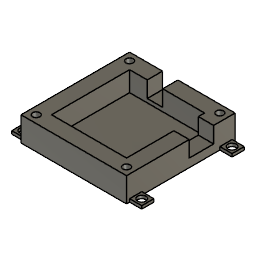
PCB_Case (Autodesk Fusion 360 archive; units mm, degrees)
design "PCB_CASE"
part number: 2026-02-23-22-04-43-512
Autodesk Fusion 360 part; units mm, degrees
sketch "Sketch1" plane through (0, 0, 0) normal (0, 0, 1) x (1, 0, 0)
  line L0 (-32.4751, 45.8669) -> (16.5249, 45.8669)
  line L1 (16.5249, 45.8669) -> (16.5249, -5.1331)
  line L2 (16.5249, -5.1331) -> (-32.4751, -5.1331)
  line L3 (-32.4751, -5.1331) -> (-32.4751, 45.8669)
  line L4 (-42.4751, 55.8669) -> (26.5249, 55.8669)
  line L5 (26.5249, 55.8669) -> (26.5249, -15.1331)
  line L6 (26.5249, -15.1331) -> (-42.4751, -15.1331)
  line L7 (-42.4751, -15.1331) -> (-42.4751, 55.8669)
  circle A0 centre (-37.4751, 50.8669) radius 2.35
  circle A1 centre (21.5249, 50.8669) radius 2.35
  circle A2 centre (-37.4751, -10.1331) radius 2.35
  circle A3 centre (21.5249, -10.1331) radius 2.35
  circle A4 centre (-37.4751, 50.8669) radius 3
  circle A5 centre (21.5249, 50.8669) radius 3
  circle A6 centre (21.5249, -10.1331) radius 3
  circle A7 centre (-37.4751, -10.1331) radius 3
  dimension "d1" = 49
  dimension "d2" = 51
  dimension "d3" = 69
  dimension "d4" = 71
  dimension "d5" = 10
  dimension "d6" = 10
  dimension "d7" = 4.7
  dimension "d8" = 4.7
  dimension "d9" = 4.7
  dimension "d10" = 4.7
  dimension "d11" = 5
  dimension "d12" = 5
  dimension "d13" = 5
  dimension "d14" = 5
  dimension "d15" = 5
  dimension "d16" = 5
  dimension "d17" = 5
  dimension "d18" = 5
  dimension "d19" = 6
  dimension "d20" = 6
  dimension "d21" = 6
  dimension "d22" = 6
  constraint horizontal L0
  constraint vertical L1
  constraint horizontal L2
  constraint vertical L3
  constraint horizontal L4
  constraint vertical L5
  constraint horizontal L6
  constraint vertical L7
  constraint concentric A0 A4
  constraint concentric A1 A5
  constraint concentric A3 A6
  constraint concentric A2 A7
  measures "d1" distance of L0.start L0.end
  measures "d2" distance of L0.start L2.end
  measures "d3" distance of L4.start L4.end
  measures "d4" distance of L4.start L6.end
  measures "d5" distance of L3 L7
  measures "d6" distance of L0 L4
  measures "d7" diameter of A0
  measures "d8" diameter of A1
  measures "d9" diameter of A2
  measures "d10" diameter of A3
  measures "d11" distance of L6 A2.centre
  measures "d12" distance of L7 A2.centre
  measures "d13" distance of L6 A3.centre
  measures "d14" distance of L5 A3.centre
  measures "d15" distance of L5 A1.centre
  measures "d16" distance of L4 A1.centre
  measures "d17" distance of L4 A0.centre
  measures "d18" distance of L7 A0.centre
  measures "d19" diameter of A4
  measures "d20" diameter of A5
  measures "d21" diameter of A6
  measures "d22" diameter of A7
extrude "Extrude1" add sketch "Sketch1" along normal blind 9.9 from surface at 3.1 contours A4 | A5 | A6 | A7 makes body 1 at (24.5211, -10.2826, 9.7) makes body 2 at (24.5211, 50.7174, 9.7) makes body 3 at (-34.4789, -10.2826, 9.7) makes body 4 at (-40.4714, 50.7174, 9.7)
extrude "Extrude2" add sketch "Sketch1" along normal blind 13 contours L4 L5 L6 L7 bodies 1 2 3 4
extrude "Extrude3" add sketch "Sketch1" along normal blind 3 contours L0 L1 L2 L3 bodies 1
sketch "Sketch2" plane through (0, 0, 13) normal (0, 0, 1) x (-1, 0, 0)
  circle A0 centre (-21.5249, 10.1331) radius 2.35
  circle A1 centre (37.4751, -50.8669) radius 2.35
  line L0 (-16.5249, 5.1331) -> (32.4751, 5.1331)
  line L1 (32.4751, 5.1331) -> (32.4751, -45.8669)
  line L2 (32.4751, -45.8669) -> (-16.5249, -45.8669)
  line L3 (-16.5249, -45.8669) -> (-16.5249, 5.1331)
  line L4 (42.4751, 15.1331) -> (-26.5249, 15.1331)
  line L5 (-26.5249, 15.1331) -> (-26.5249, -55.8669)
  line L6 (-26.5249, -55.8669) -> (42.4751, -55.8669)
  line L7 (42.4751, -55.8669) -> (42.4751, 15.1331)
  circle A2 centre (-21.5249, -50.8669) radius 2.35
  circle A3 centre (37.4751, 10.1331) radius 2.35
  line L8 (20.9211, -55.8669) -> (10.9211, -55.8669)
  line L9 (10.9211, -55.8669) -> (10.9211, -45.8669)
  line L10 (10.9211, -45.8669) -> (20.9211, -45.8669)
  line L11 (20.9211, -45.8669) -> (20.9211, -55.8669)
  line L12 (42.4751, 15.1331) -> (42.4751, -55.8669)
  line L13 (-16.5249, -41.7899) -> (-26.5249, -41.7899)
  line L14 (-26.5249, -41.7899) -> (-26.5249, -25.7899)
  line L15 (-26.5249, -25.7899) -> (-16.5249, -25.7899)
  line L16 (-16.5249, -25.7899) -> (-16.5249, -41.7899)
  line L17 (42.4751, -55.8669) -> (-26.5249, -55.8669)
  dimension "d30" = 10
  dimension "d31" = 10
  dimension "d32" = 21.554
  dimension "d33" = 10
  dimension "d34" = 16
  dimension "d35" = 14.077
  constraint horizontal L8
  constraint vertical L9
  constraint horizontal L10
  constraint vertical L11
  constraint coincident L6 L8.start
  constraint horizontal L13
  constraint vertical L14
  constraint horizontal L15
  constraint vertical L16
  constraint coincident L3 L13.start
  measures "d30" distance of L8.start L8.end
  measures "d31" distance of L8.start L10.end
  measures "d32" distance of L11 L12
  measures "d33" distance of L13.start L13.end
  measures "d34" distance of L13.start L15.end
  measures "d35" distance of L13 L17
extrude "Extrude4" cut sketch "Sketch2" against normal blind 7.5 contours L3 L5 L13 L14 L15 L16 | L2 L6 L8 L9 L10 L11 L17 bodies 1
sketch "Sketch3" plane through (0, 0, 0) normal (0, 0, 1) x (1, 0, 0)
  line L0 (-42.5221, -13.1331) -> (-50.5221, -13.1331)
  line L1 (-50.5221, -13.1331) -> (-50.5221, -5.1331)
  line L2 (-50.5221, -5.1331) -> (-42.5221, -5.1331)
  line L3 (-42.5221, -5.1331) -> (-42.5221, -13.1331)
  line L4 (26.4761, -13.1331) -> (34.4761, -13.1331)
  line L5 (34.4761, -13.1331) -> (34.4761, -5.1331)
  line L6 (34.4761, -5.1331) -> (26.4761, -5.1331)
  line L7 (26.4761, -5.1331) -> (26.4761, -13.1331)
  line L8 (26.5223, 45.8669) -> (34.5223, 45.8669)
  line L9 (34.5223, 45.8669) -> (34.5223, 53.8669)
  line L10 (34.5223, 53.8669) -> (26.5223, 53.8669)
  line L11 (26.5223, 53.8669) -> (26.5223, 45.8669)
  line L12 (-42.5, 45.8669) -> (-50.5, 45.8669)
  line L13 (-50.5, 45.8669) -> (-50.5, 53.8669)
  line L14 (-50.5, 53.8669) -> (-42.5, 53.8669)
  line L15 (-42.5, 53.8669) -> (-42.5, 45.8669)
  line L16 (26.5249, -15.1331) -> (-42.4751, -15.1331)
  line L17 (-42.4751, 55.8669) -> (26.5249, 55.8669)
  circle A0 centre (-46.5221, -9.1331) radius 2.75
  circle A1 centre (30.4761, -9.1331) radius 2.75
  circle A2 centre (30.5223, 49.8669) radius 2.75
  circle A3 centre (-46.5, 49.8669) radius 2.75
  dimension "d38" = 8
  dimension "d39" = 8
  dimension "d40" = 8
  dimension "d41" = 8
  dimension "d42" = 8
  dimension "d43" = 8
  dimension "d44" = 8
  dimension "d45" = 8
  dimension "d46" = 2
  dimension "d47" = 2
  dimension "d48" = 2
  dimension "d49" = 2
  dimension "d50" = 5.5
  dimension "d51" = 4
  dimension "d52" = 4
  dimension "d53" = 5.5
  dimension "d54" = 5.5
  dimension "d55" = 5.5
  dimension "d56" = 4
  dimension "d57" = 4
  dimension "d58" = 4
  dimension "d59" = 4
  dimension "d60" = 4
  dimension "d61" = 4
  constraint horizontal L0
  constraint vertical L1
  constraint horizontal L2
  constraint vertical L3
  constraint horizontal L4
  constraint vertical L5
  constraint horizontal L6
  constraint vertical L7
  constraint horizontal L8
  constraint vertical L9
  constraint horizontal L10
  constraint vertical L11
  constraint horizontal L12
  constraint vertical L13
  constraint horizontal L14
  constraint vertical L15
  measures "d38" distance of L0.start L0.end
  measures "d39" distance of L0.start L2.end
  measures "d40" distance of L4.start L4.end
  measures "d41" distance of L4.start L6.end
  measures "d42" distance of L8.start L8.end
  measures "d43" distance of L8.start L10.end
  measures "d44" distance of L12.start L12.end
  measures "d45" distance of L12.start L14.end
  measures "d46" distance of L0 L16
  measures "d47" distance of L4 L16
  measures "d48" distance of L10 L17
  measures "d49" distance of L14 L17
  measures "d50" diameter of A0
  measures "d51" distance of L0 A0.centre
  measures "d52" distance of L1 A0.centre
  measures "d53" diameter of A1
  measures "d54" diameter of A2
  measures "d55" diameter of A3
  measures "d56" distance of L14 A3.centre
  measures "d57" distance of L13 A3.centre
  measures "d58" distance of L10 A2.centre
  measures "d59" distance of L9 A2.centre
  measures "d60" distance of L5 A1.centre
  measures "d61" distance of L4 A1.centre
extrude "Extrude5" add sketch "Sketch3" along normal blind 2 bodies 1 makes body 5 at (-46.5685, 53.4477, 0) makes body 6 at (-46.4536, -12.7138, 0)
extrude "Extrude6" add 2 faces at (19.8582, 15.4823, 13) (-1.7725, 49.2003, 13) along direction (0, 0, 1) blind 2 on bodies 1 bodies 1
extrude "Extrude7" add 2 faces at (19.8582, 15.4823, 15) (-1.7725, 49.2003, 15) along direction (0, 0, 1) blind 1 on bodies 1 bodies 1

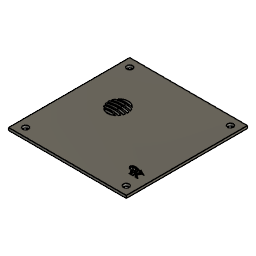
design "PCB_TOP"
part number: 2026-02-23-22-28-18-651
Autodesk Fusion 360 part; units mm, degrees
sketch "Sketch1" plane through (0, 0, 0) normal (0, 0, 1) x (1, 0, 0)
  line L0 (-55.9108, 58.924) -> (13.0892, 58.924)
  line L1 (13.0892, 58.924) -> (13.0892, -12.076)
  line L2 (13.0892, -12.076) -> (-55.9108, -12.076)
  line L3 (-55.9108, -12.076) -> (-55.9108, 58.924)
  circle A0 centre (-50.9108, 53.924) radius 1.7
  circle A1 centre (8.0892, 53.924) radius 1.7
  circle A2 centre (-50.9108, -7.076) radius 1.7
  circle A3 centre (8.0892, -7.076) radius 1.7
  dimension "d1" = 69
  dimension "d2" = 71
  dimension "d3" = 3.4
  dimension "d4" = 3.4
  dimension "d5" = 3.4
  dimension "d6" = 3.4
  dimension "d7" = 5
  dimension "d8" = 5
  dimension "d9" = 5
  dimension "d10" = 5
  dimension "d11" = 5
  dimension "d12" = 5
  dimension "d13" = 5
  dimension "d14" = 5
  constraint horizontal L0
  constraint vertical L1
  constraint horizontal L2
  constraint vertical L3
  measures "d1" distance of L0.start L0.end
  measures "d2" distance of L0.start L2.end
  measures "d3" diameter of A0
  measures "d4" diameter of A1
  measures "d5" diameter of A2
  measures "d6" diameter of A3
  measures "d7" distance of L0 A0.centre
  measures "d8" distance of L3 A0.centre
  measures "d9" distance of L0 A1.centre
  measures "d10" distance of L1 A1.centre
  measures "d11" distance of L2 A2.centre
  measures "d12" distance of L3 A2.centre
  measures "d13" distance of L1 A3.centre
  measures "d14" distance of L2 A3.centre
extrude "Extrude1" add sketch "Sketch1" along normal blind 1.5
sketch "Sketch2" plane through (0, 0, 0) normal (0, 0, -1) x (1, 0, 0)
  circle A0 centre (-50.9108, -53.924) radius 1.7
  circle A1 centre (-50.9108, 7.076) radius 1.7
  circle A2 centre (8.0892, 7.076) radius 1.7
  circle A3 centre (8.0892, -53.924) radius 1.7
  line L0 (13.0892, 12.076) -> (-55.9108, 12.076)
  line L1 (-55.9108, 12.076) -> (-55.9108, -58.924)
  line L2 (-55.9108, -58.924) -> (13.0892, -58.924)
  line L3 (13.0892, -58.924) -> (13.0892, 12.076)
sketch "Sketch3" plane through (0, 0, 0) normal (0, 0, -1) x (1, 0, 0)
sketch "Sketch4" plane through (0, 0, 0) normal (0, 0, 1) x (1, 0, 0)
  spline S0 degree 3 poles (5.6281, 1.7474) (5.8196, 2.0554) (6.0075, 2.3594) (6.1973, 2.6623) (6.3487, 2.9041) (6.502, 3.1447) (6.656, 3.3849) knots 0 0 0 0 1 1 1 2 2 2 2
  spline S1 degree 3 poles (6.656, 3.3849) (6.6671, 3.4022) (6.692, 3.4235) (6.7087, 3.422) knots 2 2 2 2 3 3 3 3
  spline S2 degree 3 poles (6.7087, 3.422) (6.7689, 3.4166) (6.8284, 3.4023) (6.9022, 3.3887) knots 3 3 3 3 4 4 4 4
  line L0 (6.9022, 3.3887) -> (5.6608, 1.7184)
  line L1 (5.6608, 1.7184) -> (5.6281, 1.7474)
  line L2 (4.5804, 1.7909) -> (4.5624, 1.7702)
  line L3 (4.5624, 1.7702) -> (5.8909, 0.5262)
  line L4 (5.8909, 0.5262) -> (5.8872, 0.5223)
  line L5 (5.8872, 0.5223) -> (4.6487, 1.4888)
  spline S3 degree 3 poles (4.6487, 1.4888) (4.6512, 1.4764) (4.6534, 1.4612) (4.6573, 1.4465) (4.7531, 1.0839) (4.8509, 0.7218) (4.9442, 0.3586) (4.9738, 0.2436) (5.0121, 0.1286) (5, 0) knots 4 4 4 4 5 5 5 6 6 6 7 7 7 7
  spline S4 degree 3 poles (5, 0) (4.9265, 0.0282) (4.8723, 0.0673) (4.8514, 0.146) (4.7035, 0.7025) (4.5538, 1.2585) (4.4057, 1.815) (4.2636, 2.3493) (4.1247, 2.8845) (3.9798, 3.4181) (3.9538, 3.5138) (3.9711, 3.5848) (4.0485, 3.6489) knots 7 7 7 7 8 8 8 9 9 9 10 10 10 11 11 11 11
  spline S5 degree 3 poles (4.0485, 3.6489) (4.057, 3.6244) (4.0653, 3.6032) (4.0716, 3.5815) (4.1522, 3.306) (4.2349, 3.0312) (4.3114, 2.7546) (4.3374, 2.6606) (4.3738, 2.584) (4.4575, 2.5237) (4.5786, 2.4365) (4.6889, 2.3342) (4.8053, 2.2373) knots 11 11 11 11 12 12 12 13 13 13 14 14 14 15 15 15 15
  line L6 (4.8053, 2.2373) -> (5.6163, 3.6354)
  line L7 (5.6163, 3.6354) -> (6.5426, 3.4546)
  line L8 (6.5426, 3.4546) -> (5.4688, 1.7209)
  spline S6 degree 3 poles (5.4688, 1.7209) (5.4886, 1.7024) (5.5045, 1.6858) (5.522, 1.6712) (5.9169, 1.3412) (6.3108, 1.0098) (6.7075, 0.682) (7.0163, 0.4267) (7.3347, 0.1848) (7.7042, 0.0204) knots 18 18 18 18 19 19 19 20 20 20 21 21 21 21
  spline S7 degree 3 poles (7.7042, 0.0204) (7.7072, 0.0191) (7.7082, 0.0133) (7.7106, 0.0087) knots 21 21 21 21 22 22 22 22
  line L9 (7.7106, 0.0087) -> (6.141, 0.0087)
  spline S8 degree 3 poles (6.141, 0.0087) (6.2596, 0.0588) (6.3866, 0.066) (6.4574, 0.1898) knots 23 23 23 23 24 24 24 24
  line L10 (6.4574, 0.1898) -> (4.5804, 1.7909)
  line L11 (3.5521, 4.7959) -> (3.5501, 4.7818)
  spline S9 degree 3 poles (3.5501, 4.7818) (3.5432, 4.7818) (3.5362, 4.7808) (3.5295, 4.782) (3.3494, 4.8151) (3.1703, 4.8556) (2.9891, 4.8801) (2.703, 4.9188) (2.4161, 4.9559) (2.1284, 4.9765) (1.9076, 4.9923) (1.6849, 4.9868) (1.4633, 4.9816) (1.1041, 4.9731) (0.7512, 4.9194) (0.4077, 4.8114) (0.1446, 4.7288) (-0.1029, 4.6155) (-0.3041, 4.4211) (-0.4819, 4.2492) (-0.586, 4.0442) (-0.565, 3.7891) (-0.5636, 3.7712) (-0.5588, 3.7537) (-0.5556, 3.736) knots 1 1 1 1 2 2 2 3 3 3 4 4 4 5 5 5 6 6 6 7 7 7 8 8 8 9 9 9 9
  spline S10 degree 3 poles (-0.5556, 3.736) (-0.5472, 3.9502) (-0.4576, 4.1249) (-0.3145, 4.276) (-0.121, 4.4805) (0.1241, 4.5996) (0.3866, 4.6832) (0.8641, 4.8353) (1.3569, 4.8719) (1.8545, 4.8528) (2.3079, 4.8355) (2.7558, 4.7693) (3.2, 4.6793) (3.7596, 4.5658) (4.3094, 4.414) (4.8543, 4.244) (4.9709, 4.2076) (5.0879, 4.1724) (5.2047, 4.1367) knots 9 9 9 9 10 10 10 11 11 11 12 12 12 13 13 13 14 14 14 15 15 15 15
  line L12 (5.2047, 4.1367) -> (5.2091, 4.1476)
  line L13 (5.2091, 4.1476) -> (3.9846, 4.702)
  spline S11 degree 3 poles (3.9846, 4.702) (4.577, 4.5581) (5.1429, 4.3403) (5.7082, 4.0808) knots 17 17 17 17 18 18 18 18
  spline S12 degree 3 poles (5.7082, 4.0808) (5.4595, 4.2577) (5.2178, 4.4195) (4.9875, 4.5961) (4.7566, 4.7731) (4.537, 4.965) (4.3124, 5.1503) knots 18 18 18 18 19 19 19 20 20 20 20
  line L14 (4.3124, 5.1503) -> (4.3217, 5.1631)
  spline S13 degree 3 poles (4.3217, 5.1631) (5.5089, 4.473) (6.7466, 3.8854) (8.0084, 3.3461) knots 21 21 21 21 22 22 22 22
  spline S14 degree 3 poles (8.0084, 3.3461) (7.662, 3.4033) (7.3162, 3.4598) (6.9722, 3.5253) (6.261, 3.6607) (5.5513, 3.8039) (4.8399, 3.9379) (4.3277, 4.0343) (3.8146, 4.1272) (3.3001, 4.2106) (2.7534, 4.2992) (2.2027, 4.345) (1.6475, 4.3283) (1.3737, 4.3201) (1.1022, 4.2966) (0.8346, 4.2389) (0.5729, 4.1826) (0.3217, 4.0989) (0.104, 3.9348) (-0.1303, 3.7584) (-0.2087, 3.495) (-0.1029, 3.2211) (-0.0226, 3.0131) (0.1228, 2.8533) (0.2889, 2.7107) (0.3566, 2.6525) (0.428, 2.5988) (0.4978, 2.5431) knots 22 22 22 22 23 23 23 24 24 24 25 25 25 26 26 26 27 27 27 28 28 28 29 29 29 30 30 30 31 31 31 31
  spline S15 degree 3 poles (0.4978, 2.5431) (0.2478, 2.6652) (0.0143, 2.8111) (-0.1869, 3.0047) (-0.3924, 3.2026) (-0.5444, 3.435) (-0.6323, 3.7066) (-0.7351, 4.0241) (-0.6754, 4.3114) (-0.4598, 4.566) (-0.3004, 4.7543) (-0.0926, 4.8718) (0.1325, 4.9605) (0.6054, 5.1469) (1.0996, 5.1935) (1.6022, 5.1694) (2.0538, 5.1477) (2.4991, 5.0781) (2.9369, 4.9649) (3.1428, 4.9117) (3.3471, 4.8524) (3.5521, 4.7959) knots 31 31 31 31 32 32 32 33 33 33 34 34 34 35 35 35 36 36 36 37 37 37 38 38 38 38
  spline S16 degree 3 poles (3.0792, 2.6831) (3.0761, 2.705) (3.0755, 2.7171) (3.0725, 2.7285) (2.998, 3.0093) (2.9217, 3.2897) (2.8492, 3.571) (2.8121, 3.7152) (2.7298, 3.8241) (2.6093, 3.9072) (2.5961, 3.9164) (2.5839, 3.9269) (2.5627, 3.9435) knots 0 0 0 0 1 1 1 2 2 2 3 3 3 4 4 4 4
  spline S17 degree 3 poles (2.5627, 3.9435) (2.5819, 3.9435) (2.5886, 3.9436) (2.5952, 3.9435) (2.8859, 3.9363) (3.1765, 3.931) (3.4671, 3.9211) (3.5886, 3.9169) (3.7097, 3.9033) (3.8222, 3.8498) (3.8726, 3.8257) (3.9161, 3.7951) (3.9397, 3.7398) knots 4 4 4 4 5 5 5 6 6 6 7 7 7 8 8 8 8
  spline S18 degree 3 poles (3.9397, 3.7398) (3.8168, 3.6538) (3.7944, 3.5454) (3.8344, 3.4021) (3.9736, 2.9036) (4.1027, 2.4022) (4.2364, 1.9021) (4.4001, 1.2897) (4.5646, 0.6775) (4.7287, 0.0652) (4.7334, 0.0475) (4.7365, 0.0294) (4.7407, 0.01) knots 8 8 8 8 9 9 9 10 10 10 11 11 11 12 12 12 12
  line L15 (4.7407, 0.01) -> (2.6293, 0.01)
  spline S19 degree 3 poles (2.6293, 0.01) (2.7311, 0.0489) (2.8207, 0.0792) (2.9069, 0.1171) (2.9939, 0.1554) (3.0751, 0.2044) (3.1385, 0.2849) knots 13 13 13 13 14 14 14 15 15 15 15
  spline S20 degree 3 poles (3.1385, 0.2849) (2.6116, 0.9618) (2.0699, 1.623) (1.5036, 2.2696) knots 15 15 15 15 16 16 16 16
  spline S21 degree 3 poles (1.5036, 2.2696) (1.5146, 2.2711) (1.5184, 2.2727) (1.5212, 2.2717) knots 16 16 16 16 17 17 17 17
  spline S22 degree 3 poles (1.5212, 2.2717) (1.8422, 2.158) (2.1718, 2.0759) (2.5055, 2.0097) (2.5464, 2.0016) (2.5744, 1.984) (2.5995, 1.9511) (2.9298, 1.5179) (3.2612, 1.0856) (3.5924, 0.6531) (3.6084, 0.6323) (3.6246, 0.6118) (3.6481, 0.5815) knots 17 17 17 17 18 18 18 19 19 19 20 20 20 21 21 21 21
  spline S23 degree 3 poles (3.6481, 0.5815) (3.6467, 0.601) (3.6472, 0.6063) (3.6459, 0.6112) (3.5264, 1.044) (3.4064, 1.4768) (3.2873, 1.9097) (3.2555, 2.025) (3.2565, 2.0238) (3.135, 2.0402) (2.6367, 2.1074) (2.1447, 2.2049) (1.6647, 2.3568) (1.3092, 2.4693) (0.9646, 2.6068) (0.6529, 2.816) (0.5076, 2.9135) (0.3678, 3.0185) (0.2641, 3.1624) (0.139, 3.3361) (0.0847, 3.5235) (0.1843, 3.7274) (0.3644, 4.0959) (0.9086, 4.1348) (1.1664, 3.7998) (1.3084, 3.6154) (1.4505, 3.4311) (1.5914, 3.246) (1.6369, 3.1862) (1.6863, 3.1346) (1.7602, 3.1086) (2.054, 3.0053) (2.3457, 2.8958) (2.641, 2.7969) (2.7817, 2.7498) (2.9286, 2.7215) (3.0792, 2.6831) knots 21 21 21 21 22 22 22 23 23 23 24 24 24 25 25 25 26 26 26 27 27 27 28 28 28 29 29 29 30 30 30 31 31 31 32 32 32 33 33 33 33
  line L16 (3.7963, 2.3959) -> (3.7953, 2.3879)
  spline S24 degree 3 poles (3.7953, 2.3879) (3.7747, 2.3879) (3.754, 2.3863) (3.7335, 2.3882) (3.5881, 2.4016) (3.4419, 2.4105) (3.2974, 2.4308) (2.7728, 2.5044) (2.2593, 2.6253) (1.7634, 2.8135) (1.4001, 2.9513) (1.0496, 3.1153) (0.7397, 3.3549) (0.6837, 3.3982) (0.6294, 3.4437) (0.5744, 3.4881) knots 1 1 1 1 2 2 2 3 3 3 4 4 4 5 5 5 6 6 6 6
  spline S25 degree 3 poles (0.5744, 3.4881) (0.5844, 3.4935) (0.5891, 3.4922) (0.593, 3.4895) knots 6 6 6 6 7 7 7 7
  spline S26 degree 3 poles (0.593, 3.4895) (0.8417, 3.32) (1.1118, 3.1913) (1.3895, 3.0786) (2.0638, 2.8049) (2.7634, 2.6158) (3.4734, 2.4622) (3.5808, 2.439) (3.6886, 2.4179) (3.7963, 2.3959) knots 7 7 7 7 8 8 8 9 9 9 10 10 10 10
  spline S27 degree 3 poles (3.0792, 2.6831) (2.9286, 2.7215) (2.7817, 2.7498) (2.641, 2.7969) (2.3457, 2.8958) (2.054, 3.0053) (1.7602, 3.1086) (1.6863, 3.1346) (1.6369, 3.1862) (1.5914, 3.246) (1.4505, 3.4311) (1.3084, 3.6154) (1.1664, 3.7998) (0.9086, 4.1348) (0.3644, 4.0959) (0.1843, 3.7274) (0.0847, 3.5235) (0.139, 3.3361) (0.2641, 3.1624) (0.3678, 3.0185) (0.5076, 2.9135) (0.6529, 2.816) (0.9646, 2.6068) (1.3092, 2.4693) (1.6647, 2.3568) (2.1447, 2.2049) (2.6367, 2.1074) (3.135, 2.0402) (3.2565, 2.0238) (3.2555, 2.025) (3.2873, 1.9097) (3.4064, 1.4768) (3.5264, 1.044) (3.6459, 0.6112) (3.6472, 0.6063) (3.6467, 0.601) (3.6481, 0.5815) knots 0 0 0 0 1 1 1 2 2 2 3 3 3 4 4 4 5 5 5 6 6 6 7 7 7 8 8 8 9 9 9 10 10 10 11 11 11 12 12 12 12
  spline S28 degree 3 poles (3.6481, 0.5815) (3.6246, 0.6118) (3.6084, 0.6323) (3.5924, 0.6531) (3.2612, 1.0856) (2.9298, 1.5179) (2.5995, 1.9511) (2.5744, 1.984) (2.5464, 2.0016) (2.5055, 2.0097) (2.1718, 2.0759) (1.8422, 2.158) (1.5212, 2.2717) knots 12 12 12 12 13 13 13 14 14 14 15 15 15 16 16 16 16
  spline S29 degree 3 poles (1.5212, 2.2717) (1.5184, 2.2727) (1.5146, 2.2711) (1.5036, 2.2696) knots 16 16 16 16 17 17 17 17
  spline S30 degree 3 poles (1.5036, 2.2696) (2.0699, 1.623) (2.6116, 0.9618) (3.1385, 0.2849) knots 17 17 17 17 18 18 18 18
  spline S31 degree 3 poles (3.1385, 0.2849) (3.0751, 0.2044) (2.9939, 0.1554) (2.9069, 0.1171) (2.8207, 0.0792) (2.7311, 0.0489) (2.6293, 0.01) knots 18 18 18 18 19 19 19 20 20 20 20
  line L17 (2.6293, 0.01) -> (4.7407, 0.01)
  spline S32 degree 3 poles (4.7407, 0.01) (4.7365, 0.0294) (4.7334, 0.0475) (4.7287, 0.0652) (4.5646, 0.6775) (4.4001, 1.2897) (4.2364, 1.9021) (4.1027, 2.4022) (3.9736, 2.9036) (3.8344, 3.4021) (3.7944, 3.5454) (3.8168, 3.6538) (3.9397, 3.7398) knots 21 21 21 21 22 22 22 23 23 23 24 24 24 25 25 25 25
  spline S33 degree 3 poles (3.9397, 3.7398) (3.9161, 3.7951) (3.8726, 3.8257) (3.8222, 3.8498) (3.7097, 3.9033) (3.5886, 3.9169) (3.4671, 3.9211) (3.1765, 3.931) (2.8859, 3.9363) (2.5952, 3.9435) (2.5886, 3.9436) (2.5819, 3.9435) (2.5627, 3.9435) knots 25 25 25 25 26 26 26 27 27 27 28 28 28 29 29 29 29
  spline S34 degree 3 poles (2.5627, 3.9435) (2.5839, 3.9269) (2.5961, 3.9164) (2.6093, 3.9072) (2.7298, 3.8241) (2.8121, 3.7152) (2.8492, 3.571) (2.9217, 3.2897) (2.998, 3.0093) (3.0725, 2.7285) (3.0755, 2.7171) (3.0761, 2.705) (3.0792, 2.6831) knots 29 29 29 29 30 30 30 31 31 31 32 32 32 33 33 33 33
  spline S35 degree 3 poles (3.5521, 4.7959) (3.3471, 4.8524) (3.1428, 4.9117) (2.9369, 4.9649) (2.4991, 5.0781) (2.0538, 5.1477) (1.6022, 5.1694) (1.0996, 5.1935) (0.6054, 5.1469) (0.1325, 4.9605) (-0.0926, 4.8718) (-0.3004, 4.7543) (-0.4598, 4.566) (-0.6754, 4.3114) (-0.7351, 4.0241) (-0.6323, 3.7066) (-0.5444, 3.435) (-0.3924, 3.2026) (-0.1869, 3.0047) (0.0143, 2.8111) (0.2478, 2.6652) (0.4978, 2.5431) knots 0 0 0 0 1 1 1 2 2 2 3 3 3 4 4 4 5 5 5 6 6 6 7 7 7 7
  spline S36 degree 3 poles (0.4978, 2.5431) (0.428, 2.5988) (0.3566, 2.6525) (0.2889, 2.7107) (0.1228, 2.8533) (-0.0226, 3.0131) (-0.1029, 3.2211) (-0.2087, 3.495) (-0.1303, 3.7584) (0.104, 3.9348) (0.3217, 4.0989) (0.5729, 4.1826) (0.8346, 4.2389) (1.1022, 4.2966) (1.3737, 4.3201) (1.6475, 4.3283) (2.2027, 4.345) (2.7534, 4.2992) (3.3001, 4.2106) (3.8146, 4.1272) (4.3277, 4.0343) (4.8399, 3.9379) (5.5513, 3.8039) (6.261, 3.6607) (6.9722, 3.5253) (7.3162, 3.4598) (7.662, 3.4033) (8.0084, 3.3461) knots 7 7 7 7 8 8 8 9 9 9 10 10 10 11 11 11 12 12 12 13 13 13 14 14 14 15 15 15 16 16 16 16
  spline S37 degree 3 poles (8.0084, 3.3461) (6.7466, 3.8854) (5.5089, 4.473) (4.3217, 5.1631) knots 16 16 16 16 17 17 17 17
  line L18 (4.3217, 5.1631) -> (4.3124, 5.1503)
  spline S38 degree 3 poles (4.3124, 5.1503) (4.537, 4.965) (4.7566, 4.7731) (4.9875, 4.5961) (5.2178, 4.4195) (5.4595, 4.2577) (5.7082, 4.0808) knots 18 18 18 18 19 19 19 20 20 20 20
  spline S39 degree 3 poles (5.7082, 4.0808) (5.1429, 4.3403) (4.577, 4.5581) (3.9846, 4.702) knots 20 20 20 20 21 21 21 21
  line L19 (3.9846, 4.702) -> (5.2091, 4.1476)
  line L20 (5.2091, 4.1476) -> (5.2047, 4.1367)
  spline S40 degree 3 poles (5.2047, 4.1367) (5.0879, 4.1724) (4.9709, 4.2076) (4.8543, 4.244) (4.3094, 4.414) (3.7596, 4.5658) (3.2, 4.6793) (2.7558, 4.7693) (2.3079, 4.8355) (1.8545, 4.8528) (1.3569, 4.8719) (0.8641, 4.8353) (0.3866, 4.6832) (0.1241, 4.5996) (-0.121, 4.4805) (-0.3145, 4.276) (-0.4576, 4.1249) (-0.5472, 3.9502) (-0.5556, 3.736) knots 23 23 23 23 24 24 24 25 25 25 26 26 26 27 27 27 28 28 28 29 29 29 29
  spline S41 degree 3 poles (-0.5556, 3.736) (-0.5588, 3.7537) (-0.5636, 3.7712) (-0.565, 3.7891) (-0.586, 4.0442) (-0.4819, 4.2492) (-0.3041, 4.4211) (-0.1029, 4.6155) (0.1446, 4.7288) (0.4077, 4.8114) (0.7512, 4.9194) (1.1041, 4.9731) (1.4633, 4.9816) (1.6849, 4.9868) (1.9076, 4.9923) (2.1284, 4.9765) (2.4161, 4.9559) (2.703, 4.9188) (2.9891, 4.8801) (3.1703, 4.8556) (3.3494, 4.8151) (3.5295, 4.782) (3.5362, 4.7808) (3.5432, 4.7818) (3.5501, 4.7818) knots 29 29 29 29 30 30 30 31 31 31 32 32 32 33 33 33 34 34 34 35 35 35 36 36 36 37 37 37 37
  line L21 (3.5501, 4.7818) -> (3.5521, 4.7959)
  line L22 (4.5804, 1.7909) -> (6.4574, 0.1898)
  spline S42 degree 3 poles (6.4574, 0.1898) (6.3866, 0.066) (6.2596, 0.0588) (6.141, 0.0087) knots 1 1 1 1 2 2 2 2
  line L23 (6.141, 0.0087) -> (7.7106, 0.0087)
  spline S43 degree 3 poles (7.7106, 0.0087) (7.7082, 0.0133) (7.7072, 0.0191) (7.7042, 0.0204) knots 3 3 3 3 4 4 4 4
  spline S44 degree 3 poles (7.7042, 0.0204) (7.3347, 0.1848) (7.0163, 0.4267) (6.7075, 0.682) (6.3108, 1.0098) (5.9169, 1.3412) (5.522, 1.6712) (5.5045, 1.6858) (5.4886, 1.7024) (5.4688, 1.7209) knots 4 4 4 4 5 5 5 6 6 6 7 7 7 7
  line L24 (5.4688, 1.7209) -> (6.5426, 3.4546)
  line L25 (6.5426, 3.4546) -> (5.6163, 3.6354)
  line L26 (5.6163, 3.6354) -> (4.8053, 2.2373)
  spline S45 degree 3 poles (4.8053, 2.2373) (4.6889, 2.3342) (4.5786, 2.4365) (4.4575, 2.5237) (4.3738, 2.584) (4.3374, 2.6606) (4.3114, 2.7546) (4.2349, 3.0312) (4.1522, 3.306) (4.0716, 3.5815) (4.0653, 3.6032) (4.057, 3.6244) (4.0485, 3.6489) knots 10 10 10 10 11 11 11 12 12 12 13 13 13 14 14 14 14
  spline S46 degree 3 poles (4.0485, 3.6489) (3.9711, 3.5848) (3.9538, 3.5138) (3.9798, 3.4181) (4.1247, 2.8845) (4.2636, 2.3493) (4.4057, 1.815) (4.5538, 1.2585) (4.7035, 0.7025) (4.8514, 0.146) (4.8723, 0.0673) (4.9265, 0.0282) (5, 0) knots 14 14 14 14 15 15 15 16 16 16 17 17 17 18 18 18 18
  spline S47 degree 3 poles (5, 0) (5.0121, 0.1286) (4.9738, 0.2436) (4.9442, 0.3586) (4.8509, 0.7218) (4.7531, 1.0839) (4.6573, 1.4465) (4.6534, 1.4612) (4.6512, 1.4764) (4.6487, 1.4888) knots 18 18 18 18 19 19 19 20 20 20 21 21 21 21
  line L27 (4.6487, 1.4888) -> (5.8872, 0.5223)
  line L28 (5.8872, 0.5223) -> (5.8909, 0.5262)
  line L29 (5.8909, 0.5262) -> (4.5624, 1.7702)
  line L30 (4.5624, 1.7702) -> (4.5804, 1.7909)
  line L31 (5.6281, 1.7474) -> (5.6608, 1.7184)
  line L32 (5.6608, 1.7184) -> (6.9022, 3.3887)
  spline S48 degree 3 poles (6.9022, 3.3887) (6.8284, 3.4023) (6.7689, 3.4166) (6.7087, 3.422) knots 2 2 2 2 3 3 3 3
  spline S49 degree 3 poles (6.7087, 3.422) (6.692, 3.4235) (6.6671, 3.4022) (6.656, 3.3849) knots 3 3 3 3 4 4 4 4
  spline S50 degree 3 poles (6.656, 3.3849) (6.502, 3.1447) (6.3487, 2.9041) (6.1973, 2.6623) (6.0075, 2.3594) (5.8196, 2.0554) (5.6281, 1.7474) knots 4 4 4 4 5 5 5 6 6 6 6
  spline S51 degree 3 poles (3.7963, 2.3959) (3.6886, 2.4179) (3.5808, 2.439) (3.4734, 2.4622) (2.7634, 2.6158) (2.0638, 2.8049) (1.3895, 3.0786) (1.1118, 3.1913) (0.8417, 3.32) (0.593, 3.4895) knots 0 0 0 0 1 1 1 2 2 2 3 3 3 3
  spline S52 degree 3 poles (0.593, 3.4895) (0.5891, 3.4922) (0.5844, 3.4935) (0.5744, 3.4881) knots 3 3 3 3 4 4 4 4
  spline S53 degree 3 poles (0.5744, 3.4881) (0.6294, 3.4437) (0.6837, 3.3982) (0.7397, 3.3549) (1.0496, 3.1153) (1.4001, 2.9513) (1.7634, 2.8135) (2.2593, 2.6253) (2.7728, 2.5044) (3.2974, 2.4308) (3.4419, 2.4105) (3.5881, 2.4016) (3.7335, 2.3882) (3.754, 2.3863) (3.7747, 2.3879) (3.7953, 2.3879) knots 4 4 4 4 5 5 5 6 6 6 7 7 7 8 8 8 9 9 9 9
  line L33 (3.7953, 2.3879) -> (3.7963, 2.3959)
extrude "Extrude2" cut sketch "Sketch4" along normal blind 1.5 contours S0 S1 S2 L0 L1 L31 L32 S48 S49 S50 | L2 L3 L4 L5 S3 S4 S5 L6 L7 L8 S6 S7 L9 S8 L10 L22 S42 L23 S43 S44 L24 L25 L26 S45 S46 S47 L27 L28 L29 L30 | L11 S9 S10 L12 L13 S11 S12 L14 S13 S14 S15 S35 S36 S37 L18 S38 S39 L19 L20 S40 S41 L21 | S16 S17 S18 L15 S19 S20 S21 S22 S23 S27 S28 S29 S30 S31 L17 S32 S33 S34 | L16 S24 S25 S26 S51 S52 S53 L33
sketch "Sketch6" plane through (0, 0, 0) normal (0, 0, -1) x (1, 0, 0)
  line L0 (5.8909, -0.5262) -> (4.5624, -1.7702)
  line L1 (4.5624, -1.7702) -> (4.5804, -1.7909)
  line L2 (4.5804, -1.7909) -> (6.4574, -0.1898)
  spline S0 degree 3 poles (6.4574, -0.1898) (6.3866, -0.066) (6.2596, -0.0588) (6.141, -0.0087) knots 1 1 1 1 2 2 2 2
  line L3 (6.141, -0.0087) -> (7.7106, -0.0087)
  spline S1 degree 3 poles (7.7106, -0.0087) (7.7082, -0.0133) (7.7072, -0.0191) (7.7042, -0.0204) knots 3 3 3 3 4 4 4 4
  spline S2 degree 3 poles (7.7042, -0.0204) (7.3347, -0.1848) (7.0163, -0.4267) (6.7075, -0.682) (6.3108, -1.0098) (5.9169, -1.3412) (5.522, -1.6712) (5.5045, -1.6858) (5.4886, -1.7024) (5.4688, -1.7209) knots 4 4 4 4 5 5 5 6 6 6 7 7 7 7
  line L4 (5.4688, -1.7209) -> (6.5426, -3.4546)
  line L5 (6.5426, -3.4546) -> (5.6163, -3.6354)
  line L6 (5.6163, -3.6354) -> (4.8053, -2.2373)
  spline S3 degree 3 poles (4.8053, -2.2373) (4.6889, -2.3342) (4.5786, -2.4365) (4.4575, -2.5237) (4.3738, -2.584) (4.3374, -2.6606) (4.3114, -2.7546) (4.2349, -3.0312) (4.1522, -3.306) (4.0716, -3.5815) (4.0653, -3.6032) (4.057, -3.6244) (4.0485, -3.6489) knots 10 10 10 10 11 11 11 12 12 12 13 13 13 14 14 14 14
  spline S4 degree 3 poles (4.0485, -3.6489) (3.9711, -3.5848) (3.9538, -3.5138) (3.9798, -3.4181) (4.1247, -2.8845) (4.2636, -2.3493) (4.4057, -1.815) (4.5538, -1.2585) (4.7035, -0.7025) (4.8514, -0.146) (4.8723, -0.0673) (4.9265, -0.0282) (5, 0) knots 14 14 14 14 15 15 15 16 16 16 17 17 17 18 18 18 18
  spline S5 degree 3 poles (5, 0) (5.0121, -0.1286) (4.9738, -0.2436) (4.9442, -0.3586) (4.8509, -0.7218) (4.7531, -1.0839) (4.6573, -1.4465) (4.6534, -1.4612) (4.6512, -1.4764) (4.6487, -1.4888) knots 18 18 18 18 19 19 19 20 20 20 21 21 21 21
  line L7 (4.6487, -1.4888) -> (5.8872, -0.5223)
  line L8 (5.8872, -0.5223) -> (5.8909, -0.5262)
  spline S6 degree 3 poles (-0.5556, -3.736) (-0.5588, -3.7537) (-0.5636, -3.7712) (-0.565, -3.7891) (-0.586, -4.0442) (-0.4819, -4.2492) (-0.3041, -4.4211) (-0.1029, -4.6155) (0.1446, -4.7288) (0.4077, -4.8114) (0.7512, -4.9194) (1.1041, -4.9731) (1.4633, -4.9816) (1.6849, -4.9868) (1.9076, -4.9923) (2.1284, -4.9765) (2.4161, -4.9559) (2.703, -4.9188) (2.9891, -4.8801) (3.1703, -4.8556) (3.3494, -4.8151) (3.5295, -4.782) (3.5362, -4.7808) (3.5432, -4.7818) (3.5501, -4.7818) knots 29 29 29 29 30 30 30 31 31 31 32 32 32 33 33 33 34 34 34 35 35 35 36 36 36 37 37 37 37
  line L9 (3.5501, -4.7818) -> (3.5521, -4.7959)
  spline S7 degree 3 poles (3.5521, -4.7959) (3.3471, -4.8524) (3.1428, -4.9117) (2.9369, -4.9649) (2.4991, -5.0781) (2.0538, -5.1477) (1.6022, -5.1694) (1.0996, -5.1935) (0.6054, -5.1469) (0.1325, -4.9605) (-0.0926, -4.8718) (-0.3004, -4.7543) (-0.4598, -4.566) (-0.6754, -4.3114) (-0.7351, -4.0241) (-0.6323, -3.7066) (-0.5444, -3.435) (-0.3924, -3.2026) (-0.1869, -3.0047) (0.0143, -2.8111) (0.2478, -2.6652) (0.4978, -2.5431) knots 0 0 0 0 1 1 1 2 2 2 3 3 3 4 4 4 5 5 5 6 6 6 7 7 7 7
  spline S8 degree 3 poles (0.4978, -2.5431) (0.428, -2.5988) (0.3566, -2.6525) (0.2889, -2.7107) (0.1228, -2.8533) (-0.0226, -3.0131) (-0.1029, -3.2211) (-0.2087, -3.495) (-0.1303, -3.7584) (0.104, -3.9348) (0.3217, -4.0989) (0.5729, -4.1826) (0.8346, -4.2389) (1.1022, -4.2966) (1.3737, -4.3201) (1.6475, -4.3283) (2.2027, -4.345) (2.7534, -4.2992) (3.3001, -4.2106) (3.8146, -4.1272) (4.3277, -4.0343) (4.8399, -3.9379) (5.5513, -3.8039) (6.261, -3.6607) (6.9722, -3.5253) (7.3162, -3.4598) (7.662, -3.4033) (8.0084, -3.3461) knots 7 7 7 7 8 8 8 9 9 9 10 10 10 11 11 11 12 12 12 13 13 13 14 14 14 15 15 15 16 16 16 16
  spline S9 degree 3 poles (8.0084, -3.3461) (6.7466, -3.8854) (5.5089, -4.473) (4.3217, -5.1631) knots 16 16 16 16 17 17 17 17
  line L10 (4.3217, -5.1631) -> (4.3124, -5.1503)
  spline S10 degree 3 poles (4.3124, -5.1503) (4.537, -4.965) (4.7566, -4.7731) (4.9875, -4.5961) (5.2178, -4.4195) (5.4595, -4.2577) (5.7082, -4.0808) knots 18 18 18 18 19 19 19 20 20 20 20
  spline S11 degree 3 poles (5.7082, -4.0808) (5.1429, -4.3403) (4.577, -4.5581) (3.9846, -4.702) knots 20 20 20 20 21 21 21 21
  line L11 (3.9846, -4.702) -> (5.2091, -4.1476)
  line L12 (5.2091, -4.1476) -> (5.2047, -4.1367)
  spline S12 degree 3 poles (5.2047, -4.1367) (5.0879, -4.1724) (4.9709, -4.2076) (4.8543, -4.244) (4.3094, -4.414) (3.7596, -4.5658) (3.2, -4.6793) (2.7558, -4.7693) (2.3079, -4.8355) (1.8545, -4.8528) (1.3569, -4.8719) (0.8641, -4.8353) (0.3866, -4.6832) (0.1241, -4.5996) (-0.121, -4.4805) (-0.3145, -4.276) (-0.4576, -4.1249) (-0.5472, -3.9502) (-0.5556, -3.736) knots 23 23 23 23 24 24 24 25 25 25 26 26 26 27 27 27 28 28 28 29 29 29 29
  spline S13 degree 3 poles (3.9397, -3.7398) (3.9161, -3.7951) (3.8726, -3.8257) (3.8222, -3.8498) (3.7097, -3.9033) (3.5886, -3.9169) (3.4671, -3.9211) (3.1765, -3.931) (2.8859, -3.9363) (2.5952, -3.9435) (2.5886, -3.9436) (2.5819, -3.9435) (2.5627, -3.9435) knots 25 25 25 25 26 26 26 27 27 27 28 28 28 29 29 29 29
  spline S14 degree 3 poles (2.5627, -3.9435) (2.5839, -3.9269) (2.5961, -3.9164) (2.6093, -3.9072) (2.7298, -3.8241) (2.8121, -3.7152) (2.8492, -3.571) (2.9217, -3.2897) (2.998, -3.0093) (3.0725, -2.7285) (3.0755, -2.7171) (3.0761, -2.705) (3.0792, -2.6831) knots 29 29 29 29 30 30 30 31 31 31 32 32 32 33 33 33 33
  spline S15 degree 3 poles (3.0792, -2.6831) (2.9286, -2.7215) (2.7817, -2.7498) (2.641, -2.7969) (2.3457, -2.8958) (2.054, -3.0053) (1.7602, -3.1086) (1.6863, -3.1346) (1.6369, -3.1862) (1.5914, -3.246) (1.4505, -3.4311) (1.3084, -3.6154) (1.1664, -3.7998) (0.9086, -4.1348) (0.3644, -4.0959) (0.1843, -3.7274) (0.0847, -3.5235) (0.139, -3.3361) (0.2641, -3.1624) (0.3678, -3.0185) (0.5076, -2.9135) (0.6529, -2.816) (0.9646, -2.6068) (1.3092, -2.4693) (1.6647, -2.3568) (2.1447, -2.2049) (2.6367, -2.1074) (3.135, -2.0402) (3.2565, -2.0238) (3.2555, -2.025) (3.2873, -1.9097) (3.4064, -1.4768) (3.5264, -1.044) (3.6459, -0.6112) (3.6472, -0.6063) (3.6467, -0.601) (3.6481, -0.5815) knots 0 0 0 0 1 1 1 2 2 2 3 3 3 4 4 4 5 5 5 6 6 6 7 7 7 8 8 8 9 9 9 10 10 10 11 11 11 12 12 12 12
  spline S16 degree 3 poles (3.6481, -0.5815) (3.6246, -0.6118) (3.6084, -0.6323) (3.5924, -0.6531) (3.2612, -1.0856) (2.9298, -1.5179) (2.5995, -1.9511) (2.5744, -1.984) (2.5464, -2.0016) (2.5055, -2.0097) (2.1718, -2.0759) (1.8422, -2.158) (1.5212, -2.2717) knots 12 12 12 12 13 13 13 14 14 14 15 15 15 16 16 16 16
  spline S17 degree 3 poles (1.5212, -2.2717) (1.5184, -2.2727) (1.5146, -2.2711) (1.5036, -2.2696) knots 16 16 16 16 17 17 17 17
  spline S18 degree 3 poles (1.5036, -2.2696) (2.0699, -1.623) (2.6116, -0.9618) (3.1385, -0.2849) knots 17 17 17 17 18 18 18 18
  spline S19 degree 3 poles (3.1385, -0.2849) (3.0751, -0.2044) (2.9939, -0.1554) (2.9069, -0.1171) (2.8207, -0.0792) (2.7311, -0.0489) (2.6293, -0.01) knots 18 18 18 18 19 19 19 20 20 20 20
  line L13 (2.6293, -0.01) -> (4.7407, -0.01)
  spline S20 degree 3 poles (4.7407, -0.01) (4.7365, -0.0294) (4.7334, -0.0475) (4.7287, -0.0652) (4.5646, -0.6775) (4.4001, -1.2897) (4.2364, -1.9021) (4.1027, -2.4022) (3.9736, -2.9036) (3.8344, -3.4021) (3.7944, -3.5454) (3.8168, -3.6538) (3.9397, -3.7398) knots 21 21 21 21 22 22 22 23 23 23 24 24 24 25 25 25 25
  spline S21 degree 3 poles (6.7087, -3.422) (6.692, -3.4235) (6.6671, -3.4022) (6.656, -3.3849) knots 3 3 3 3 4 4 4 4
  spline S22 degree 3 poles (6.656, -3.3849) (6.502, -3.1447) (6.3487, -2.9041) (6.1973, -2.6623) (6.0075, -2.3594) (5.8196, -2.0554) (5.6281, -1.7474) knots 4 4 4 4 5 5 5 6 6 6 6
  line L14 (5.6281, -1.7474) -> (5.6608, -1.7184)
  line L15 (5.6608, -1.7184) -> (6.9022, -3.3887)
  spline S23 degree 3 poles (6.9022, -3.3887) (6.8284, -3.4023) (6.7689, -3.4166) (6.7087, -3.422) knots 2 2 2 2 3 3 3 3
  circle A0 centre (-50.9108, -53.924) radius 1.7
  circle A1 centre (-50.9108, 7.076) radius 1.7
  circle A2 centre (8.0892, 7.076) radius 1.7
  circle A3 centre (8.0892, -53.924) radius 1.7
  line L16 (13.0892, 12.076) -> (-55.9108, 12.076)
  line L17 (-55.9108, 12.076) -> (-55.9108, -58.924)
  line L18 (-55.9108, -58.924) -> (13.0892, -58.924)
  line L19 (13.0892, -58.924) -> (13.0892, 12.076)
  spline S24 degree 3 poles (-30.673, -25.4383) (-31.9156, -24.4277) (-33.3073, -24.0112) (-34.856, -24.1921) (-35.7885, -24.301) (-37.4438, -25.038) (-37.655, -25.4626) knots 0 0 0 0 1 1 1 2 2 2 2
  spline S25 degree 3 poles (-37.655, -25.4626) (-35.3226, -25.9794) (-32.9995, -25.9962) (-30.673, -25.4383) knots 2 2 2 2 3 3 3 3
  spline S26 degree 3 poles (-30.0204, -34.4621) (-31.3862, -34.8059) (-32.7665, -34.9737) (-34.1663, -34.9697) (-35.5634, -34.9658) (-36.9415, -34.7912) (-38.3062, -34.4602) knots 0 0 0 0 1 1 1 2 2 2 2
  spline S27 degree 3 poles (-38.3062, -34.4602) (-37.2147, -35.657) (-35.9005, -36.3333) (-34.3341, -36.3779) (-32.6373, -36.4262) (-31.2052, -35.7562) (-30.0204, -34.4621) knots 2 2 2 2 3 3 3 4 4 4 4
  spline S28 degree 3 poles (-39.1279, -27.1588) (-39.0567, -27.1905) (-39.0126, -27.2152) (-38.9658, -27.2302) (-37.7899, -27.6071) (-36.5879, -27.8276) (-35.3642, -27.9203) (-33.7757, -28.0407) (-32.2011, -27.9378) (-30.6442, -27.5759) (-30.1997, -27.4726) (-29.7614, -27.3387) (-29.32, -27.2198) (-29.2379, -27.1976) (-29.206, -27.1595) (-29.2654, -27.076) (-29.4747, -26.7815) (-29.6832, -26.4864) (-29.8916, -26.1912) (-29.9449, -26.1157) (-30.0053, -26.0953) (-30.0966, -26.1215) (-30.9248, -26.3596) (-31.7664, -26.5243) (-32.6203, -26.6074) (-33.4848, -26.6916) (-34.3507, -26.707) (-35.2179, -26.6402) (-36.2521, -26.5606) (-37.2725, -26.3964) (-38.2753, -26.1113) (-38.3092, -26.1016) (-38.3651, -26.1186) (-38.3897, -26.1453) (-38.4832, -26.2472) (-38.5742, -26.3532) (-38.655, -26.4667) (-38.812, -26.6875) (-38.9616, -26.9144) (-39.1279, -27.1588) knots 0 0 0 0 1 1 1 2 2 2 3 3 3 4 4 4 5 5 5 6 6 6 7 7 7 8 8 8 9 9 9 10 10 10 11 11 11 12 12 12 13 13 13 13
  spline S29 degree 3 poles (-33.9274, -34.1489) (-33.4107, -34.1507) (-32.6896, -34.1071) (-31.971, -34.0131) (-31.072, -33.8956) (-30.1875, -33.701) (-29.315, -33.4429) knots 0 0 0 0 1 1 1 2 2 2 2
  spline S30 degree 3 poles (-29.315, -33.4429) (-29.2801, -33.4326) (-29.241, -33.4028) (-29.2227, -33.37) (-29.0131, -32.9942) (-28.8419, -32.5991) (-28.7182, -32.1814) (-28.7069, -32.1433) (-28.7134, -32.0991) (-28.7116, -32.0578) knots 2 2 2 2 3 3 3 4 4 4 5 5 5 5
  spline S31 degree 3 poles (-28.7116, -32.0578) (-28.7503, -32.0592) (-28.7914, -32.0517) (-28.8271, -32.0633) knots 5 5 5 5 6 6 6 6
  spline S32 degree 3 poles (-28.8271, -32.0633) (-30.1133, -32.4796) (-31.4241, -32.7502) (-32.7655, -32.8549) (-34.0141, -32.9524) (-35.2588, -32.9181) (-36.4995, -32.7504) (-37.5203, -32.6124) (-38.5248, -32.3858) (-39.508, -32.0566) (-39.5394, -32.0461) (-39.5922, -32.043) (-39.6079, -32.062) knots 6 6 6 6 7 7 7 8 8 8 9 9 9 10 10 10 10
  spline S33 degree 3 poles (-39.6079, -32.062) (-39.6253, -32.0832) (-39.6223, -32.1386) (-39.6097, -32.1708) (-39.4832, -32.4949) (-39.3494, -32.8158) (-39.2249, -33.1408) (-39.1461, -33.3464) (-39.0156, -33.4439) (-38.8081, -33.5012) (-37.2744, -33.9247) (-35.7194, -34.1562) (-33.9274, -34.1489) knots 10 10 10 10 11 11 11 12 12 12 13 13 13 14 14 14 14
  spline S34 degree 3 poles (-33.9581, -30.0252) (-33.1916, -30.02) (-32.2255, -29.9497) (-31.2665, -29.7815) (-30.3697, -29.6241) (-29.4907, -29.3893) (-28.6255, -29.0925) (-28.5615, -29.0705) (-28.5301, -29.0403) (-28.5509, -28.9674) (-28.644, -28.6417) (-28.7373, -28.3161) (-28.8303, -27.9904) (-28.8526, -27.912) (-28.8894, -27.8942) (-28.968, -27.9215) (-30.5091, -28.4571) (-32.0913, -28.7402) (-33.7098, -28.7877) (-34.5879, -28.8134) (-35.4628, -28.7588) (-36.3345, -28.6392) (-37.3559, -28.4992) (-38.3592, -28.2732) (-39.338, -27.9289) (-39.4224, -27.8991) (-39.4657, -27.9118) (-39.4918, -28.0029) (-39.5799, -28.3108) (-39.6676, -28.6189) (-39.7609, -28.925) (-39.7924, -29.0282) (-39.7683, -29.0703) (-39.6701, -29.1046) (-37.8802, -29.729) (-36.0431, -30.0258) (-33.9581, -30.0252) knots 0 0 0 0 1 1 1 2 2 2 3 3 3 4 4 4 5 5 5 6 6 6 7 7 7 8 8 8 9 9 9 10 10 10 11 11 11 12 12 12 12
  spline S35 degree 3 poles (-34.0803, -32.0825) (-33.1166, -32.0877) (-32.2131, -32.0053) (-31.3148, -31.8545) (-30.3868, -31.6987) (-29.4757, -31.4669) (-28.5818, -31.1568) (-28.5063, -31.1306) (-28.4661, -31.0934) (-28.463, -31.0056) (-28.4514, -30.6759) (-28.4332, -30.3465) (-28.4239, -30.0168) (-28.4197, -29.8683) (-28.4521, -29.8492) (-28.5848, -29.8965) (-29.8738, -30.3555) (-31.1958, -30.6469) (-32.5484, -30.774) (-33.9777, -30.9083) (-35.4032, -30.8627) (-36.8228, -30.6378) (-37.8105, -30.4813) (-38.7809, -30.2452) (-39.7263, -29.8978) (-39.8643, -29.8472) (-39.8989, -29.8703) (-39.8951, -30.0322) (-39.8883, -30.329) (-39.875, -30.6257) (-39.8607, -30.9222) (-39.8511, -31.1233) (-39.8478, -31.1218) (-39.6708, -31.1826) (-38.6249, -31.5419) (-37.556, -31.7914) (-36.467, -31.9401) (-35.6571, -32.0507) (-34.8433, -32.1007) (-34.0803, -32.0825) knots 0 0 0 0 1 1 1 2 2 2 3 3 3 4 4 4 5 5 5 6 6 6 7 7 7 8 8 8 9 9 9 10 10 10 11 11 11 12 12 12 13 13 13 13
  spline S36 degree 3 poles (-34.0803, -32.0825) (-34.8433, -32.1007) (-35.6571, -32.0507) (-36.467, -31.9401) (-37.556, -31.7914) (-38.6249, -31.5419) (-39.6708, -31.1826) (-39.8478, -31.1218) (-39.8511, -31.1233) (-39.8607, -30.9222) (-39.875, -30.6257) (-39.8883, -30.329) (-39.8951, -30.0322) (-39.8989, -29.8703) (-39.8643, -29.8472) (-39.7263, -29.8978) (-38.7809, -30.2452) (-37.8105, -30.4813) (-36.8228, -30.6378) (-35.4032, -30.8627) (-33.9777, -30.9083) (-32.5484, -30.774) (-31.1958, -30.6469) (-29.8738, -30.3555) (-28.5848, -29.8965) (-28.4521, -29.8492) (-28.4197, -29.8683) (-28.4239, -30.0168) (-28.4332, -30.3465) (-28.4514, -30.6759) (-28.463, -31.0056) (-28.4661, -31.0934) (-28.5063, -31.1306) (-28.5818, -31.1568) (-29.4757, -31.4669) (-30.3868, -31.6987) (-31.3148, -31.8545) (-32.2131, -32.0053) (-33.1166, -32.0877) (-34.0803, -32.0825) knots 0 0 0 0 1 1 1 2 2 2 3 3 3 4 4 4 5 5 5 6 6 6 7 7 7 8 8 8 9 9 9 10 10 10 11 11 11 12 12 12 13 13 13 13
  spline S37 degree 3 poles (-33.9581, -30.0252) (-36.0431, -30.0258) (-37.8802, -29.729) (-39.6701, -29.1046) (-39.7683, -29.0703) (-39.7924, -29.0282) (-39.7609, -28.925) (-39.6676, -28.6189) (-39.5799, -28.3108) (-39.4918, -28.0029) (-39.4657, -27.9118) (-39.4224, -27.8991) (-39.338, -27.9289) (-38.3592, -28.2732) (-37.3559, -28.4992) (-36.3345, -28.6392) (-35.4628, -28.7588) (-34.5879, -28.8134) (-33.7098, -28.7877) (-32.0913, -28.7402) (-30.5091, -28.4571) (-28.968, -27.9215) (-28.8894, -27.8942) (-28.8526, -27.912) (-28.8303, -27.9904) (-28.7373, -28.3161) (-28.644, -28.6417) (-28.5509, -28.9674) (-28.5301, -29.0403) (-28.5615, -29.0705) (-28.6255, -29.0925) (-29.4907, -29.3893) (-30.3697, -29.6241) (-31.2665, -29.7815) (-32.2255, -29.9497) (-33.1916, -30.02) (-33.9581, -30.0252) knots 0 0 0 0 1 1 1 2 2 2 3 3 3 4 4 4 5 5 5 6 6 6 7 7 7 8 8 8 9 9 9 10 10 10 11 11 11 12 12 12 12
  spline S38 degree 3 poles (-33.9274, -34.1489) (-35.7194, -34.1562) (-37.2744, -33.9247) (-38.8081, -33.5012) (-39.0156, -33.4439) (-39.1461, -33.3464) (-39.2249, -33.1408) (-39.3494, -32.8158) (-39.4832, -32.4949) (-39.6097, -32.1708) (-39.6223, -32.1386) (-39.6253, -32.0832) (-39.6079, -32.062) knots 0 0 0 0 1 1 1 2 2 2 3 3 3 4 4 4 4
  spline S39 degree 3 poles (-39.6079, -32.062) (-39.5922, -32.043) (-39.5394, -32.0461) (-39.508, -32.0566) (-38.5248, -32.3858) (-37.5203, -32.6124) (-36.4995, -32.7504) (-35.2588, -32.9181) (-34.0141, -32.9524) (-32.7655, -32.8549) (-31.4241, -32.7502) (-30.1133, -32.4796) (-28.8271, -32.0633) knots 4 4 4 4 5 5 5 6 6 6 7 7 7 8 8 8 8
  spline S40 degree 3 poles (-28.8271, -32.0633) (-28.7914, -32.0517) (-28.7503, -32.0592) (-28.7116, -32.0578) knots 8 8 8 8 9 9 9 9
  spline S41 degree 3 poles (-28.7116, -32.0578) (-28.7134, -32.0991) (-28.7069, -32.1433) (-28.7182, -32.1814) (-28.8419, -32.5991) (-29.0131, -32.9942) (-29.2227, -33.37) (-29.241, -33.4028) (-29.2801, -33.4326) (-29.315, -33.4429) knots 9 9 9 9 10 10 10 11 11 11 12 12 12 12
  spline S42 degree 3 poles (-29.315, -33.4429) (-30.1875, -33.701) (-31.072, -33.8956) (-31.971, -34.0131) (-32.6896, -34.1071) (-33.4107, -34.1507) (-33.9274, -34.1489) knots 12 12 12 12 13 13 13 14 14 14 14
  spline S43 degree 3 poles (-39.1279, -27.1588) (-38.9616, -26.9144) (-38.812, -26.6875) (-38.655, -26.4667) (-38.5742, -26.3532) (-38.4832, -26.2472) (-38.3897, -26.1453) (-38.3651, -26.1186) (-38.3092, -26.1016) (-38.2753, -26.1113) (-37.2725, -26.3964) (-36.2521, -26.5606) (-35.2179, -26.6402) (-34.3507, -26.707) (-33.4848, -26.6916) (-32.6203, -26.6074) (-31.7664, -26.5243) (-30.9248, -26.3596) (-30.0966, -26.1215) (-30.0053, -26.0953) (-29.9449, -26.1157) (-29.8916, -26.1912) (-29.6832, -26.4864) (-29.4747, -26.7815) (-29.2654, -27.076) (-29.206, -27.1595) (-29.2379, -27.1976) (-29.32, -27.2198) (-29.7614, -27.3387) (-30.1997, -27.4726) (-30.6442, -27.5759) (-32.2011, -27.9378) (-33.7757, -28.0407) (-35.3642, -27.9203) (-36.5879, -27.8276) (-37.7899, -27.6071) (-38.9658, -27.2302) (-39.0126, -27.2152) (-39.0567, -27.1905) (-39.1279, -27.1588) knots 0 0 0 0 1 1 1 2 2 2 3 3 3 4 4 4 5 5 5 6 6 6 7 7 7 8 8 8 9 9 9 10 10 10 11 11 11 12 12 12 13 13 13 13
  spline S44 degree 3 poles (-30.0204, -34.4621) (-31.2052, -35.7562) (-32.6373, -36.4262) (-34.3341, -36.3779) (-35.9005, -36.3333) (-37.2147, -35.657) (-38.3062, -34.4602) knots 0 0 0 0 1 1 1 2 2 2 2
  spline S45 degree 3 poles (-38.3062, -34.4602) (-36.9415, -34.7912) (-35.5634, -34.9658) (-34.1663, -34.9697) (-32.7665, -34.9737) (-31.3862, -34.8059) (-30.0204, -34.4621) knots 2 2 2 2 3 3 3 4 4 4 4
  spline S46 degree 3 poles (-30.673, -25.4383) (-32.9995, -25.9962) (-35.3226, -25.9794) (-37.655, -25.4626) knots 0 0 0 0 1 1 1 1
  spline S47 degree 3 poles (-37.655, -25.4626) (-37.4438, -25.038) (-35.7885, -24.301) (-34.856, -24.1921) (-33.3073, -24.0112) (-31.9156, -24.4277) (-30.673, -25.4383) knots 1 1 1 1 2 2 2 3 3 3 3
extrude "Extrude3" cut sketch "Sketch6" against normal blind 1.5 contours S24 S25 S46 S47 | S26 S27 S44 S45 | S28 S43 | S29 S30 S31 S32 S33 S38 S39 S40 S41 S42 | S34 S37 | S35 S36
